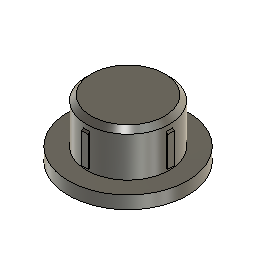
rod_end_cap (Autodesk Fusion 360 design; units mm, degrees)
part number: 2026-09-03-23-52-10-226
Autodesk Fusion 360 part; units mm, degrees
sketch "End cap profile" plane through (0, 0, 0) normal (0, 1, 0) x (1, 0, 0)
  line L0 (0, 0) -> (18.7, 0)
  line L1 (18.7, 0) -> (18.7, -4)
  line L2 (18.7, -4) -> (13, -4)
  line L3 (13, -4) -> (13, -16.5)
  line L4 (13, -16.5) -> (11.5, -18)
  line L5 (11.5, -18) -> (0, -18)
  line L6 (0, -18) -> (0, 0)
  dimension "d11" = 18.7
  dimension "d12" = 4
  dimension "d13" = 13
  dimension "d14" = 18
  dimension "d15" = 1.5
  dimension "d16" = 1.5
  constraint horizontal L0
  constraint horizontal L2
  constraint horizontal L5
  constraint vertical L1
  constraint vertical L3
  constraint vertical L6
  constraint coincident L0.start L6.end
  measures "d11" horizontal distance of L0.start L0.end
  measures "d12" vertical distance of L0.end L1.end
  measures "d13" horizontal distance of L0.start L2.end
  measures "d14" vertical distance of L0.start L5.end
  measures "d15" horizontal distance of L3.end L4.end
  measures "d16" vertical distance of L3.end L4.end
revolve "End cap revolve" add sketch "End cap profile" angle 360 about axis through (0, 0, 1.75) along (0, 0, 1)
sketch "Crush rib" plane through (0, 0, 0) normal (0, 1, 0) x (1, 0, 0)
  line L0 (12, -5) -> (13.5, -5)
  line L1 (13.5, -5) -> (13.5, -14.5)
  line L2 (13.5, -14.5) -> (12, -16)
  line L3 (12, -16) -> (12, -5)
  dimension "d18" = 12
  dimension "d19" = 5
  dimension "d20" = 13.5
  dimension "d21" = 16
  dimension "d22" = 14.5
  constraint horizontal L0
  constraint vertical L1
  constraint vertical L3
  measures "d18" horizontal distance of origin L0.start
  measures "d19" vertical distance of origin L0.start
  measures "d20" horizontal distance of origin L0.end
  measures "d21" vertical distance of origin L2.end
  measures "d22" vertical distance of origin L1.end
extrude "Crush rib (1)" add sketch "Crush rib" along normal mid plane 2
pattern_circular "Crush ribs" count 4 over 360 about axis through (0, 0, 1.75) along (0, 0, 1) of "Crush rib (1)"
equation "rodOuterDiameter = 33.4 mm" comment "drives the model; safe to edit live in Fusion"
equation "pipeInnerDiameter = 26.6 mm" comment "drives the model; safe to edit live in Fusion"
equation "endCapFlangeProud = 2.0 mm" comment "drives the model; safe to edit live in Fusion"
equation "endCapFlangeThickness = 4.0 mm" comment "drives the model; safe to edit live in Fusion"
equation "endCapStemLength = 14.0 mm" comment "drives the model; safe to edit live in Fusion"
equation "endCapStemDiameter = pipeInnerDiameter - 0.6 mm" comment "drives the model; safe to edit live in Fusion"
equation "endCapRibDiameter = pipeInnerDiameter + 0.4 mm" comment "drives the model; safe to edit live in Fusion"
equation "endCapTipChamfer = 1.5 mm" comment "drives the model; safe to edit live in Fusion"
equation "endCapRibWidth = 2.0 mm" comment "drives the model; safe to edit live in Fusion"
equation "endCapRibCount = 4" comment "drives the model; safe to edit live in Fusion"
equation "d11 = rodOuterDiameter / 2 + endCapFlangeProud"
equation "d12 = endCapFlangeThickness"
equation "d13 = endCapStemDiameter / 2"
equation "d14 = endCapFlangeThickness + endCapStemLength"
equation "d15 = endCapTipChamfer"
equation "d16 = endCapTipChamfer"
equation "d18 = endCapStemDiameter / 2 - 1 mm"
equation "d19 = endCapFlangeThickness + 1 mm"
equation "d20 = endCapRibDiameter / 2"
equation "d21 = endCapFlangeThickness + endCapStemLength - 2 mm"
equation "d22 = endCapFlangeThickness + endCapStemLength - 3.5 mm"
equation "d23 = endCapRibWidth"
equation "d25 = endCapRibCount"
named bodies: "rod_end_cap"
